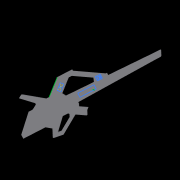
# Autodesk Inventor part: Hybrid
Saved by Autodesk Inventor 2020 (Build 240168000, 168)
## iProperties
Created: 2022-11-06
Part Number: Hybrid
Material: Generic
Document SubType Name: Modeling
Designer: Val
Density: 1 g/cm^3
Appearance: Default
Author: Val
Autodesk Inventor part; units mm, degrees
ref_plane "YZ Plane" through (0, 0, 0) normal (1, 0, 0) x (0, 1, 0)
ref_plane "XZ Plane" through (0, 0, 0) normal (0, 1, 0) x (-1, 0, 0)
ref_plane "XY Plane" through (0, 0, 0) normal (0, 0, 1) x (1, 0, 0)
sketch "SteinbergBoden5" plane through (0, 0, 0) normal (0, 0, 1) x (1, 0, 0)
  line L0 (-265.1838, 66.2948) -> (610.5672, 45.41)
  line L1 (-253.4935, -33.7986) -> (584.2, -11.1347)
  line L2 (610.5672, 45.41) -> (584.2, -11.1347)
  line L3 (-1044.1237, 0) -> (1819.7424, 0) construction
  line L4 (-265.1838, 66.2948) -> (-253.4935, -33.7986) construction
  line L5 (-330.2, 8551.4827) -> (-370.5371, 8546.5299)
  line L6 (-370.5371, 8546.5299) -> (-353.5119, 8407.8713)
  line L7 (-353.5119, 8407.8713) -> (-313.1749, 8412.824)
  line L8 (-313.1749, 8412.824) -> (-330.2, 8551.4827)
  line L9 (0, -2467.2392) -> (0, 8195.2792) construction
  line L10 (-442.9271, 4255.2831) -> (-482.3599, 4245.4514)
  line L11 (-482.3599, 4245.4514) -> (-448.5634, 4109.901)
  line L12 (-448.5634, 4109.901) -> (-409.1306, 4119.7327)
  line L13 (-409.1306, 4119.7327) -> (-442.9271, 4255.2831)
  line L14 (-612.775, 70.027) -> (-533.4, 70.027)
  line L15 (-533.4, 70.027) -> (-533.4, 52.247) construction
  line L16 (-533.4, 52.247) -> (-612.775, 52.247)
  line L17 (-612.775, 52.247) -> (-612.775, 70.027)
  circle A0 centre (-533.4, 61.137) radius 8.89
  line L18 (-612.775, 70.027) -> (-630.555, 70.027)
  line L19 (-630.555, 70.027) -> (-630.555, 52.247)
  line L20 (-630.555, 52.247) -> (-612.775, 52.247)
  line L21 (-612.775, 52.247) -> (-612.775, 70.027)
  line L22 (-533.4, 61.137) -> (-477.9163, -57.8481) construction
  line L23 (-635, 228.6) -> (0, 228.6) construction
  line L24 (0, 228.6) -> (0, -209.55) construction
  line L25 (0, -209.55) -> (-635, -209.55) construction
  line L26 (-635, -209.55) -> (-635, 228.6) construction
  line L27 (610.5672, 45.41) -> (643.2113, 45.41)
  line L28 (643.2113, 45.41) -> (643.2113, -1224.5469)
  line L29 (643.2113, -1224.5469) -> (1641.3825, -11.1347)
  line L30 (1641.3825, -11.1347) -> (584.2, -11.1347)
  line L31 (-533.4, 61.137) -> (623.244, 37.4869) construction
  line L32 (-523.2994, 39.4761) -> (616.4636, 35.647) construction
  line L33 (-508.4047, 7.5344) -> (611.3127, 14.4361) construction
  line L34 (-490.4999, -30.8625) -> (605.289, -9.6889) construction
  line L35 (-474.5383, -65.0923) -> (600.1336, -32.0278) construction
  circle A1 centre (-523.2994, 39.4761) radius 8.89
  circle A2 centre (-508.4047, 7.5344) radius 8.89
  circle A3 centre (-490.4999, -30.8625) radius 8.89
  circle A4 centre (-474.5383, -65.0923) radius 8.89
  circle A5 centre (-337.8933, -92.7495) radius 12.7
  line L36 (0, 203.2) -> (-635, 203.2) construction
  line L37 (-635, 203.2) -> (-635, -158.75) construction
  line L38 (-635, -158.75) -> (0, -158.75) construction
  line L39 (0, -158.75) -> (0, 203.2) construction
  line L40 (-635, -127) -> (0, -127) construction
  line L41 (0, -127) -> (0, 152.4) construction
  line L42 (0, 152.4) -> (-635, 152.4) construction
  line L43 (-635, 152.4) -> (-635, -127) construction
  line L44 (-523.2994, 48.3661) -> (-602.6744, 48.3661)
  line L45 (-602.6744, 48.3661) -> (-602.6744, 30.5861)
  line L46 (-602.6744, 30.5861) -> (-523.2994, 30.5861)
  line L47 (-523.2994, 30.5861) -> (-523.2994, 48.3661) construction
  line L48 (-602.6744, 48.3661) -> (-620.4544, 48.3661)
  line L49 (-620.4544, 48.3661) -> (-620.4544, 30.5861)
  line L50 (-620.4544, 30.5861) -> (-602.6744, 30.5861)
  line L51 (-602.6744, 30.5861) -> (-602.6744, 48.3661)
  line L52 (-508.4047, 16.4244) -> (-587.7797, 16.4244)
  line L53 (-587.7797, 16.4244) -> (-587.7797, -1.3556)
  line L54 (-587.7797, -1.3556) -> (-508.4047, -1.3556)
  line L55 (-508.4047, -1.3556) -> (-508.4047, 16.4244) construction
  line L56 (-587.7797, 16.4244) -> (-605.5597, 16.4244)
  line L57 (-605.5597, 16.4244) -> (-605.5597, -1.3556)
  line L58 (-605.5597, -1.3556) -> (-587.7797, -1.3556)
  line L59 (-587.7797, -1.3556) -> (-587.7797, 16.4244)
  line L60 (-490.4999, -21.9725) -> (-569.8749, -21.9725)
  line L61 (-569.8749, -21.9725) -> (-569.8749, -39.7525)
  line L62 (-569.8749, -39.7525) -> (-490.4999, -39.7525)
  line L63 (-490.4999, -39.7525) -> (-490.4999, -21.9725) construction
  line L64 (-569.8749, -21.9725) -> (-587.6549, -21.9725)
  line L65 (-587.6549, -21.9725) -> (-587.6549, -39.7525)
  line L66 (-587.6549, -39.7525) -> (-569.8749, -39.7525)
  line L67 (-569.8749, -39.7525) -> (-569.8749, -21.9725)
  line L68 (-474.5383, -56.2023) -> (-553.9133, -56.2023)
  line L69 (-553.9133, -56.2023) -> (-553.9133, -73.9823)
  line L70 (-553.9133, -73.9823) -> (-474.5383, -73.9823)
  line L71 (-474.5383, -73.9823) -> (-474.5383, -56.2023)
  line L72 (-553.9133, -56.2023) -> (-571.6933, -56.2023)
  line L73 (-571.6933, -56.2023) -> (-571.6933, -73.9823)
  line L74 (-571.6933, -73.9823) -> (-553.9133, -73.9823)
  line L75 (-553.9133, -73.9823) -> (-553.9133, -56.2023)
  point P0 (0, 0)
  dimension "d0" = 876
  dimension "d1" = 838
  dimension "d2" = 115
  dimension "d3" = 584.2
  dimension "d4" = 7
  dimension "d5" = 139.7
  dimension "d6" = 40.64
  dimension "d7" = 14
  dimension "d8" = 17.78
  dimension "d9" = 17.78
  dimension "d10" = 79.375
  dimension "d11" = 25.4
  dimension "d12" = 635
  dimension "d13" = 330.2
  dimension "d14" = 72.39
  dimension "d15" = 533.4
  dimension "d16" = 25
  dimension "d17" = 25.4
  dimension "d18" = 50.8
  dimension "d19" = 152.4
  dimension "d20" = 127
  dimension "d21" = 31.75
  dimension "d22" = 50.8
  dimension "d23" = 91.366
  dimension "d24" = 91.55
  dimension "d25" = 39.441
  dimension "d26" = 88.238
  dimension "d27" = 88.893
  dimension "d28" = 90.353
  dimension "d29" = 89.808
  dimension "d30" = 88.829
  dimension "d31" = 6.662
  dimension "d32" = 70.027
  dimension "d33" = 643.2113
  dimension "d34" = 45.41
  dimension "d35" = 130.6695
  dimension "d36" = 5.4935
  dimension "d37" = 13.775
  dimension "d38" = 21.8843
  dimension "d39" = 31.6042
  dimension "d40" = 1091.7534
  dimension "d41" = 1166.0124
  dimension "d42" = 623.244
  dimension "d43" = 616.4636
  dimension "d44" = 611.3127
  dimension "d45" = 605.289
  dimension "d46" = 600.1336
  dimension "d47" = 337.8933
  dimension "d48" = 92.7495
  dimension "d49" = 477.9163
  constraints: 148 end point, 31 parallel, 18 perpendicular, 14 horizontal, 10 equal length, 8 collinear, 8 point on circle, 6 centre point, 5 point on line, 5 tangent, 4 coincident, 4 equal radius, 1 midpoint
  measures "d0" distance of L0.start L0.end
  measures "d1" distance of L1.start L1.end
  measures "d2" angle of L2 L3
  measures "d3" horizontal distance of L1.end point (0, 0)
  measures "d4" angle of L8 L9
  measures "d5" distance of L7.end L5.start
  measures "d6" distance of L5.start L5.end
  measures "d7" angle of L9 L13
  measures "d8" distance of L16.end L14.start
  measures "d9" distance between parallel lines of L17 L19
  measures "d10" distance of L14.start L14.end
  measures "d11" diameter of A5
  measures "d12" distance of L23.start L23.end
  measures "d13" distance from line of L5.start L9
  measures "d14" horizontal distance of L10.start L5.end
  measures "d15" distance from line of L9 L22.start
  measures "d16" angle of L43 L22
  measures "d17" distance between parallel lines of L36 L23
  measures "d18" distance between parallel lines of L42 L36
  measures "d19" distance between parallel lines of L3 L42
  measures "d20" distance from line of point (0, 0) L40
  measures "d21" distance between parallel lines of L38 L40
  measures "d22" distance between parallel lines of L25 L38
  measures "d23" angle of L9 L0
  measures "d24" angle of L24 L1
  measures "d25" angle of L29 L9
  measures "d26" angle of L35 L9
  measures "d27" angle of L34 L9
  measures "d28" angle of L33 L9
  measures "d29" angle of L32 L9
  measures "d30" angle of L31 L9
  measures "d31" angle of L4 L9
  measures "d32" distance between parallel lines of L3 L14
  measures "d33" distance between parallel lines of L28 L9
  measures "d34" distance between parallel lines of L27 L3
  measures "d35" distance from line of L3.end L29
  measures "d36" distance from line of L3.end L35
  measures "d37" distance from line of L3.end L34
  measures "d38" distance from line of L3.end L33
  measures "d39" distance from line of L3.end L32
  measures "d40" distance from line of L3.end L8
  measures "d41" distance from line of L3.end L13
  measures "d42" distance from line of L31.end L9
  measures "d43" distance from line of L32.end L9
  measures "d44" distance from line of L33.end L9
  measures "d45" distance from line of L34.end L9
  measures "d46" distance from line of L35.end L9
  measures "d47" distance from line of A5.centre L9
  measures "d48" distance from line of A5.centre L3
  measures "d49" distance from line of L22.end L9
sketch "Base" plane through (0, 0, 0) normal (0, 0, 1) x (1, 0, 0)
  line L0 (-265.1838, 66.2948) -> (610.5672, 45.41) projected
  line L1 (-253.4935, -33.7986) -> (584.2, -11.1347) projected
  line L2 (-630.555, 70.027) -> (-630.555, 52.247) projected
  line L3 (-612.775, 70.027) -> (-630.555, 70.027) projected
  line L4 (-630.555, 52.247) -> (-612.775, 52.247) projected
  line L5 (-612.775, 52.247) -> (-612.775, 70.027) projected
  line L6 (-612.775, 70.027) -> (-533.4, 70.027) projected
  line L7 (-533.4, 52.247) -> (-612.775, 52.247) projected
  circle A0 centre (-533.4, 61.137) radius 8.89 projected
  circle A1 centre (-523.2994, 39.4761) radius 8.89 projected
  line L8 (-523.2994, 48.3661) -> (-602.6744, 48.3661) projected
  line L9 (-602.6744, 30.5861) -> (-523.2994, 30.5861) projected
  line L10 (-602.6744, 48.3661) -> (-602.6744, 30.5861) projected
  line L11 (-602.6744, 48.3661) -> (-620.4544, 48.3661) projected
  line L12 (-620.4544, 30.5861) -> (-602.6744, 30.5861) projected
  line L13 (-620.4544, 48.3661) -> (-620.4544, 30.5861) projected
  line L14 (-605.5597, 16.4244) -> (-605.5597, -1.3556) projected
  line L15 (-587.7797, 16.4244) -> (-605.5597, 16.4244) projected
  line L16 (-605.5597, -1.3556) -> (-587.7797, -1.3556) projected
  line L17 (-508.4047, 16.4244) -> (-587.7797, 16.4244) projected
  line L18 (-587.7797, -1.3556) -> (-508.4047, -1.3556) projected
  circle A2 centre (-508.4047, 7.5344) radius 8.89 projected
  circle A3 centre (-490.4999, -30.8625) radius 8.89 projected
  circle A4 centre (-474.5383, -65.0923) radius 8.89 projected
  line L19 (-490.4999, -21.9725) -> (-569.8749, -21.9725) projected
  line L20 (-569.8749, -39.7525) -> (-490.4999, -39.7525) projected
  line L21 (-569.8749, -21.9725) -> (-569.8749, -39.7525) projected
  line L22 (-569.8749, -21.9725) -> (-587.6549, -21.9725) projected
  line L23 (-587.6549, -39.7525) -> (-569.8749, -39.7525) projected
  line L24 (-587.6549, -21.9725) -> (-587.6549, -39.7525) projected
  line L25 (-571.6933, -56.2023) -> (-571.6933, -73.9823) projected
  line L26 (-553.9133, -56.2023) -> (-571.6933, -56.2023) projected
  line L27 (-571.6933, -73.9823) -> (-553.9133, -73.9823) projected
  line L28 (-553.9133, -73.9823) -> (-474.5383, -73.9823) projected
  line L29 (-474.5383, -56.2023) -> (-553.9133, -56.2023) projected
  line L30 (-533.4, 61.137) -> (623.244, 37.4869) construction
  line L31 (-523.2994, 39.4761) -> (616.4636, 35.647) construction
  line L32 (-508.4047, 7.5344) -> (611.3127, 14.4361) construction
  line L33 (-490.4999, -30.8625) -> (605.289, -9.6889) construction
  line L34 (-474.5383, -65.0923) -> (600.1336, -32.0278) construction
  line L35 (-587.7797, -1.3556) -> (-587.7797, 16.4244) projected
  line L36 (-553.9133, -56.2023) -> (-553.9133, -73.9823) projected
  line L37 (-302.7546, -14.2759) -> (-288.4229, -34.7436)
  line L38 (-253.4935, -33.7986) -> (-288.4229, -34.7436)
  line L39 (-265.1838, 66.2948) -> (-302.7546, -14.2759)
  line L40 (-249.8117, 99.3456) -> (-231.3256, 65.4874)
  line L41 (-249.8117, 99.3456) -> (-139.6504, 193.8782)
  line L42 (-361.5717, 119.38) -> (-390.1467, 119.38)
  line L43 (-361.5717, 119.38) -> (-224.4383, 237.0582)
  line L44 (-224.4383, 237.0582) -> (-89.3317, 237.0582)
  line L45 (-1138.5252, 0) -> (1835.476, 0) construction
  line L46 (-139.6504, 193.8782) -> (-111.0754, 193.8782)
  line L47 (-111.0754, 193.8782) -> (46.8805, 95.1764)
  line L48 (-89.3317, 237.0582) -> (166.2104, 77.3778) construction
  line L49 (46.8805, 95.1764) -> (33.7735, 59.1653)
  line L50 (610.5672, 45.41) -> (584.2, -11.1347)
  line L51 (-139.6504, 193.8782) -> (-89.3317, 237.0582) construction
  line L52 (-390.1467, 119.38) -> (-557.5007, 245.4903)
  line L53 (-482.3599, 87.8141) -> (-480.3469, 87.8141)
  line L54 (-531.8838, 88.9) -> (-569.9838, 88.9)
  line L55 (-569.9838, 88.9) -> (-713.6679, -54.7841)
  line L56 (-713.6679, -54.7841) -> (-713.6679, -92.8841)
  line L57 (-456.7922, -128.5466) -> (-491.6793, -203.3623)
  line L58 (-491.6793, -203.3623) -> (-397.4756, -217.4411)
  line L59 (-397.4756, -217.4411) -> (-230.5373, -113.1265)
  line L60 (-553.9133, 76.1812) -> (-553.9133, -73.9823)
  line L61 (-553.9133, -73.9823) -> (-557.7886, -80.1841)
  line L62 (-557.7886, -80.1841) -> (-631.1179, -80.1841)
  line L63 (-631.1179, -80.1841) -> (-631.1179, 27.7659)
  line L64 (-631.1179, 27.7659) -> (-568.3079, 90.5759)
  line L65 (-568.3079, 90.5759) -> (-553.9133, 76.1812)
  line L66 (-487.8897, 114.3) -> (-531.8838, 88.9)
  line L67 (-713.6679, -92.8841) -> (-504.1179, -92.8841)
  line L68 (-504.1179, -92.8841) -> (-456.7922, -128.5466)
  line L69 (-553.9133, 76.1812) -> (-531.8838, 88.9) construction
  line L70 (-487.8897, 114.3) -> (-487.8897, 127)
  line L71 (-557.5007, 245.4903) -> (-590.4963, 226.4403)
  line L72 (-487.8897, 127) -> (-590.4963, 226.4403)
  line L73 (-163.0546, -31.3518) -> (-163.0546, -44.0518)
  line L74 (-163.0546, -44.0518) -> (-173.7891, -67.072)
  line L75 (-173.7891, -67.072) -> (-106.4752, -109.1343)
  line L76 (-230.5373, -113.1265) -> (-144.8632, -166.6617)
  line L77 (-125.751, -125.6754) -> (-144.8632, -166.6617)
  line L78 (-106.4752, -109.1343) -> (-125.751, -125.6754)
  line L79 (166.2104, 77.3778) -> (165.701, 56.0191)
  line L80 (610.5672, 45.41) -> (661.3672, 45.41)
  line L81 (584.2, -11.1347) -> (635, -11.1347)
  line L82 (661.3672, 45.41) -> (635, -11.1347)
  line L83 (-89.3317, 237.0582) -> (-80.8735, 237.0582)
  line L84 (-80.8735, 237.0582) -> (-80.8735, 224.3582)
  line L85 (-80.8735, 224.3582) -> (154.3443, 77.3778)
  line L86 (154.3443, 77.3778) -> (166.2104, 77.3778)
  line L87 (-284.4959, -109.4047) -> (-273.8634, -86.6032)
  line L88 (-273.8634, -86.6032) -> (-281.1479, -76.2)
  line L89 (-281.1479, -76.2) -> (-335.5425, -76.2)
  line L90 (-335.5425, -76.2) -> (-428.2379, -172.1889)
  line L91 (-428.2379, -172.1889) -> (-429.4881, -180.5542)
  line L92 (-429.4881, -180.5542) -> (-404.3671, -184.3086)
  line L93 (-404.3671, -184.3086) -> (-284.4959, -109.4047)
  point P0 (0, 0)
  dimension "d51" = 88.9
  dimension "d54" = 33.8582
  dimension "d55" = 120
  dimension "d56" = 102
  dimension "d57" = 119.38
  dimension "d58" = 33.8582
  dimension "d59" = 237.0582
  dimension "d60" = 43.18
  dimension "d61" = 148
  dimension "d62" = 28.575
  dimension "d63" = 186.2582
  dimension "d64" = 120.65
  dimension "d65" = 102
  dimension "d66" = 28.575
  dimension "d67" = 111.76
  dimension "d68" = 143
  dimension "d70" = 209.55
  dimension "d73" = 50.8
  dimension "d74" = 30
  dimension "d75" = 38.1
  dimension "d76" = 88.9
  dimension "d77" = 45
  dimension "d78" = 38.1
  dimension "d80" = 304.8
  dimension "d81" = 209.55
  dimension "d82" = 203.2
  dimension "d83" = 59.2582
  dimension "d84" = 115
  dimension "d85" = 82.55
  dimension "d86" = 8.5
  dimension "d87" = 32
  dimension "d88" = 95.25
  dimension "d89" = 196.85
  dimension "d93" = 120
  dimension "d94" = 82.55
  dimension "d95" = 12.7
  dimension "d96" = 38.1
  dimension "d97" = 12.7
  dimension "d98" = 139.7
  dimension "d99" = 12.7
  dimension "d100" = 25.4
  dimension "d101" = 79.375
  dimension "d102" = 25.4
  dimension "d104" = 50.8
  dimension "d105" = 8.4582
  dimension "d106" = 12.7
  dimension "d107" = 122
  dimension "d113" = 31.75
  dimension "d114" = 31.75
  dimension "d115" = 50.8
  dimension "d116" = 76.2
  dimension "d117" = 12.7
  dimension "d118" = 8.4582
  dimension "d119" = 14
  dimension "d120" = 25.4
  constraints: 112 end point, 24 parallel, 6 horizontal, 5 collinear, 4 perpendicular, 4 point on line, 3 vertical
  measures "d51" distance of L0.start L37.start
  measures "d54" horizontal distance of L0.start L40.end
  measures "d55" angle of L0 L40
  measures "d56" angle of L41 L40
  measures "d57" distance between parallel lines of L45 L42
  measures "d58" vertical distance of L40.end L40.start
  measures "d59" distance between parallel lines of L44 L45
  measures "d60" distance between parallel lines of L44 L46
  measures "d61" angle of L47 L46
  measures "d62" distance of L46.end L41.end
  measures "d63" distance of L46.end L47.end
  measures "d64" distance of L47.end L48.end
  measures "d65" angle of L47 L49
  measures "d66" distance of L42.start L42.end
  measures "d67" horizontal distance of L40.start L42.start
  measures "d68" angle of L52 L42
  measures "d70" distance of L42.end L52.end
  measures "d73" distance of L66.start L54.start
  measures "d74" angle of L45 L66
  measures "d75" distance of L54.start L54.end
  measures "d76" distance between parallel lines of L45 L54
  measures "d77" angle of L45 L55
  measures "d78" distance of L55.end L56.end
  measures "d80" horizontal distance of L0.start L54.end
  measures "d81" distance of L56.end L67.end
  measures "d82" distance of L54.end L55.end
  measures "d83" distance of L67.end L57.start
  measures "d84" angle of L45 L39
  measures "d85" distance of L57.start L57.end
  measures "d86" angle of L58 L45
  measures "d87" angle of L45 L59
  measures "d88" distance of L57.end L58.end
  measures "d89" distance of L58.end L59.end
  measures "d93" angle of L39 L37
  measures "d94" distance between parallel lines of L56 L63
  measures "d95" distance between parallel lines of L67 L62
  measures "d96" distance of L52.end L71.end
  measures "d97" distance of L66.start L70.end
  measures "d98" horizontal distance of L37.start L73.start
  measures "d99" distance of L73.start L73.end
  measures "d100" distance of L73.end L74.end
  measures "d101" distance of L74.end L75.end
  measures "d102" distance of L75.end L77.start
  measures "d104" distance of L0.end L80.end
  measures "d105" distance of L44.end L83.end
  measures "d106" distance of L83.end L84.end
  measures "d107" angle of L61 L62
  measures "d113" distance between parallel lines of L59 L93
  measures "d114" distance between parallel lines of L58 L92
  measures "d115" distance of L59.end L87.end
  measures "d116" distance between parallel lines of L45 L89
  measures "d117" distance of L87.end L88.end
  measures "d118" distance of L90.end L91.end
  measures "d119" angle of L93 L90
  measures "d120" distance of L91.end L92.end
extrude "Extrusion1" add sketch "Base" along normal blind 50.8 contours L39 L37 L38 L1 L73 L74 L75 L78 L77 L76 L59 L58 L57 L68 L67 L56 L55 L63 L62 L61 L28 A4 L29 L60 L20 A3 L19 L18 A2 L17 L9 A1 L8 L7 A0 L6 L65 L54 L66 L70 L72 L71 L52 L42 L43 L44 L83 L84 L85 L86 L79 L0 L49 L47 L46 L41 L40 | L0 L50 L1 L38 L37 L39 | L80 L82 L81 L50 | L65 L60 L6 L55 L54 | L55 L13 L12 L9 L60 L17 L15 L14 L16 L18 L19 L22 L24 L23 L20 L26 L25 L27 L61 L62 L63 | L55 L11 L10 L12 L13 | L6 L60 L7 L55 | L6 A0 L7 L60 | L55 L7 L60 L8 L11 | A0 | L10 L8 L60 L9 | L36 L29 A4 L28 | L27 L25 L26 L36 | L8 A1 L9 L60 | A4 | A1 | L60 L18 L35 L17 | L17 A2 L18 L60 | L60 L19 A3 L20 | L20 L21 L19 L60 | A2 | L35 L16 L14 L15 | L23 L24 L22 L21 | A3
chamfer "Chamfer1" distance 6.35 angle 45 2 edges at (-144.8632, -166.6617, 25.4) (-491.6793, -203.3623, 25.4)
chamfer "Chamfer3" distance 6.35 angle 45 2 edges at (661.3672, 45.41, 25.4) (635, -11.1347, 25.4)
sketch "Sketch3" plane through (0, 0, 50.8) normal (0, 0, 1) x (1, 0, 0)
  line L0 (61.9125, 95.1764) -> (109.5375, 95.1764)
  line L1 (109.5375, 95.1764) -> (109.5375, 55.5625)
  line L2 (109.5375, 55.5625) -> (61.9125, 55.5625)
  line L3 (61.9125, 55.5625) -> (61.9125, 95.1764)
  line L4 (72.848, 85.725) -> (88.9, 85.725)
  line L5 (88.9, 85.725) -> (88.9, 63.5)
  line L6 (88.9, 63.5) -> (72.848, 63.5)
  line L7 (72.848, 63.5) -> (72.848, 85.725)
  line L8 (95.25, 85.725) -> (101.6, 85.725)
  line L9 (101.6, 85.725) -> (101.6, 63.5)
  line L10 (101.6, 63.5) -> (95.25, 63.5)
  line L11 (95.25, 63.5) -> (95.25, 85.725)
  line L12 (-224.4383, 237.0582) -> (-361.5717, 119.38) projected
  line L13 (-274.5728, 138.9125) -> (-222.2284, 185.2164)
  line L14 (-222.2284, 185.2164) -> (-200.2197, 160.3365)
  line L15 (-200.2197, 160.3365) -> (-252.5641, 114.0326)
  line L16 (-252.5641, 114.0326) -> (-274.5728, 138.9125)
  line L17 (-274.5728, 138.9125) -> (-200.2197, 160.3365) construction
  line L18 (-222.2284, 185.2164) -> (-252.5641, 114.0326) construction
  line L19 (-131.7625, 39.6875) -> (22.225, 39.6875)
  line L20 (22.225, 39.6875) -> (22.225, 0)
  line L21 (22.225, 0) -> (-131.7625, 0)
  line L22 (-131.7625, 0) -> (-131.7625, 39.6875)
  point P0 (0, 0)
  point P1 (-237.3962, 149.6245)
  constraints: 44 end point, 10 parallel, 5 perpendicular, 4 horizontal, 2 midpoint
body "Solid1"
